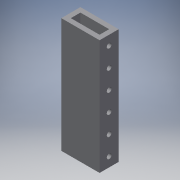
# Autodesk Inventor part: Front Frame
Saved by Autodesk Inventor 2017 (Build 210142000, 142)
## iProperties
Created: 2017-12-29
Part Number: Front Frame
Material: Generic
Document SubType Name: Modeling
Designer: anikasoojin
Density: 1 g/cm^3
Appearance: Default
Author: anikasoojin
Autodesk Inventor part; units mm, degrees
ref_plane "YZ Plane" through (0, 0, 0) normal (1, 0, 0) x (0, 1, 0)
ref_plane "XZ Plane" through (0, 0, 0) normal (0, 1, 0) x (-1, 0, 0)
ref_plane "XY Plane" through (0, 0, 0) normal (0, 0, 1) x (1, 0, 0)
sketch "Sketch1" plane through (0, 0, 0) normal (0, 1, 0) x (-1, 0, 0)
  line L0 (-24.2371, 7.8342) -> (26.5629, 7.8342)
  line L1 (26.5629, 7.8342) -> (26.5629, 33.2342)
  line L2 (26.5629, 33.2342) -> (-24.2371, 33.2342)
  line L3 (-24.2371, 33.2342) -> (-24.2371, 7.8342)
  line L4 (-17.8871, 14.1842) -> (20.2129, 14.1842)
  line L5 (20.2129, 14.1842) -> (20.2129, 26.8842)
  line L6 (20.2129, 26.8842) -> (-17.8871, 26.8842)
  line L7 (-17.8871, 26.8842) -> (-17.8871, 14.1842)
  point P0 (0, 0)
  dimension "d0" = 50.8
  dimension "d1" = 25.4
  dimension "d2" = 6.35
  constraints: 16 end point, 4 parallel, 2 perpendicular, 1 horizontal, 3 other
  measures "d0" distance of L1.end L2.end
  measures "d1" distance of L2.end L0.start
  measures "d2" distance between parallel lines of L3 L7
extrude "Extrusion1" add sketch "Sketch1" along normal blind 152.4
sketch "Sketch2" plane through (24.2371, 0, 33.2342) normal (1, 0, 0) x (0, 0, -1)
  line L0 (19.05, 0) -> (6.35, 0) projected
  line L1 (12.7, 0) -> (12.7, 152.4) construction
  line L2 (6.35, 152.4) -> (19.05, 152.4) projected
  circle A0 centre (12.7, 12.7) radius 3.175
  circle A1 centre (12.7, 38.1) radius 3.175
  circle A2 centre (12.7, 63.5) radius 3.175
  circle A3 centre (12.7, 88.9) radius 3.175
  circle A4 centre (12.7, 114.3) radius 3.175
  circle A5 centre (12.7, 139.7) radius 3.175
  point P0 (33.2342, 0)
  dimension "d5" = 6.35
  dimension "d6" = 12.7
  dimension "d9" = 25.4
  constraints: 6 centre point, 2 end point, 2 midpoint, 1 point on line, 1 vertical, 10 other
  measures "d5" diameter of A0
  measures "d6" distance from line of L0 A0.centre
  measures "d9" distance of A0.centre A1.centre
extrude "Extrusion2" cut sketch "Sketch2" against normal through all
body "Solid1"
